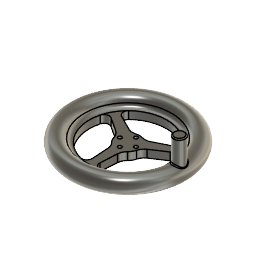
New+Assembly (Autodesk Fusion 360 archive; units mm, degrees)
design "handle"
Autodesk Fusion 360 part; units mm, degrees
note: some values were not read from the file. Set by a fixed rule: the direction of a hole.
sketch "Sketch1" plane through (0, 0, 0) normal (0, 1, 0) x (1, 0, 0)
  line L0 (0, 0) -> (50.8, 0)
  circle A0 centre (50.8, -8.255) radius 8.255
  line L1 (38.2276, -7.62) -> (0, -7.62)
  line L2 (0, -7.62) -> (0, 0)
  arc A1 (43.0171, -11.0067) -> (38.2276, -7.62) centre (38.2276, -12.7) ccw
  line L3 (45.085, -14.2118) -> (56.515, -14.2118)
  line L4 (56.515, -14.2118) -> (56.515, -39.6118)
  line L5 (56.515, -39.6118) -> (45.085, -39.6118)
  line L6 (45.085, -39.6118) -> (45.085, -14.2118)
  line L7 (50.8, -39.6118) -> (50.8, -14.2118)
  dimension "d1" = 16.51
  dimension "d2" = 7.62
  dimension "d3" = 5.08
  dimension "d4" = 50.8
  dimension "d6" = 25.4
  dimension "d20" = 11.43
  constraint coincident L0.start L2.end
  constraint horizontal L0
  constraint horizontal L1
  constraint vertical L2
  constraint tangent L0 A0
  constraint coincident L0.end A0
  constraint tangent A0 A1
  constraint coincident A0 A1.start
  constraint tangent L1 A1
  constraint horizontal L3
  constraint vertical L4
  constraint horizontal L5
  constraint vertical L6
  constraint coincident A0 L3.start
  constraint coincident A0 L3.end
  constraint midpoint L5 L7.start
  constraint midpoint L3 L7.end
  measures "d1" diameter of A0
  measures "d2" distance of L1.end L0.start
  measures "d3" radius of A1
  measures "d4" distance of A0.centre L2
  measures "d6" distance of L3.end L4.end
  measures "d20" distance of L3.start L3.end
revolve "Revolve1" add sketch "Sketch1" angle 360 about axis through (0, 0, 7.62) along (0, 0, -1) contours L0 A0 L1 L2 A1 | A0 L3 | A0 L3 L7 | A0 L3 L7
revolve "Revolve2" add sketch "Sketch1" angle 360 about axis through (50.8, 0, 39.6118) along (0, 0, -1) contours A0 L4 L5 L7 | A0 L3 L7 picked at (51.1497, -15.7216)
sketch "Sketch2" plane through (0, 0, 0) normal (0, 0, -1) x (1, 0, 0)
  circle A0 centre (0, 0) radius 50.8
  line L0 (0, 0) -> (50.8, 0)
  circle A1 centre (0, 0) radius 11.5
  circle A2 centre (0, 0) radius 38.2276
  line L1 (-5.08, 10.3172) -> (-3.429, 38.0735)
  line L2 (3.429, 38.0735) -> (5.08, 10.3172)
  line L3 (0, 0) -> (0, 8) construction
  line L4 (-6.3949, -9.558) -> (-31.2582, -22.0064)
  line L5 (-34.6872, -16.0672) -> (-11.4749, -0.7592)
  line L6 (11.4749, -0.7592) -> (34.6872, -16.0672)
  line L7 (31.2582, -22.0064) -> (6.3949, -9.558)
  point P0 (8, 0)
  point P1 (0, 8)
  point P2 (-8, 0)
  point P3 (0, -8)
  dimension "d9" = 8
  dimension "d11" = 360
  dimension "d12" = 23
  dimension "d13" = 6.858
  dimension "d14" = 10.16
  dimension "d16" = 360
  constraint coincident P0 L0
  constraint coincident A0.centre L0.start
  constraint coincident A1 L1.start
  constraint coincident A2 L1.end
  constraint coincident A2 L2.start
  constraint coincident P1 L3.end
  constraint symmetric L1 L2 L3
  constraint coincident A1 L2.end
  measures "d9" distance of P0 A0.centre
  measures "d12" diameter of A1
  measures "d13" distance of L1.end L2.start
  measures "d14" distance of L1.start L2.end
extrude "Extrude1" cut sketch "Sketch2" against normal through all contours L0 A1 A2 L2 | L0 A1 A2 L6 | A1 A2 L1 L5 | A1 A2 L4 L7
hole "Hole1" at (-8, 0, 0) at (0, -8, 0) at (8, 0, 0) at (0, 8, 0) direction (0, 0, 1) diameter 3.5992 end through all
fillet "Fillet1" radius 5.08 6 edges at (-34.6872, 16.0672, 3.81) (-31.2582, 22.0064, 3.81) (34.6872, 16.0672, 3.81) (31.2582, 22.0064, 3.81) (-3.429, -38.0735, 3.81) (3.429, -38.0735, 3.81)
fillet "Fillet1" radius 10.16 6 edges at (5.08, -10.3172, 3.81) (-5.08, -10.3172, 3.81) (-11.4749, 0.7592, 3.81) (-6.3949, 9.558, 3.81) (11.4749, 0.7592, 3.81) (6.3949, 9.558, 3.81)
fillet "Fillet1" radius 1.016 1 edges at (45.4717, -2.0666, 39.6118)
fillet "Fillet1" radius 1.016 2 edges at (50.6592, -5.7133, 16.508) (50.6414, 5.7128, 16.5084)

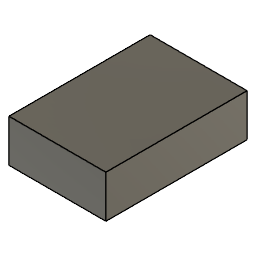
design "bread board w/ pico vol"
Autodesk Fusion 360 part; units mm, degrees
sketch "Sketch1" plane through (0, 0, 0) normal (0, 0, 1) x (1, 0, 0)
  line L0 (0, 0) -> (57, 0)
  line L1 (57, 0) -> (57, 83)
  line L2 (57, 83) -> (0, 83)
  line L3 (0, 83) -> (0, 0)
  dimension "d1" = 57
  dimension "d2" = 83
  constraint horizontal L0
  constraint vertical L1
  constraint horizontal L2
  constraint vertical L3
  constraint coincident L0.start L3.end
  measures "d1" distance of L0.start L0.end
  measures "d2" distance of L0.start L2.end
extrude "Extrude1" add sketch "Sketch1" along normal blind 25

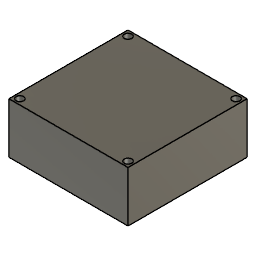
design "driver vol"
Autodesk Fusion 360 part; units mm, degrees
sketch "Sketch1" plane through (0, 0, 0) normal (0, 0, 1) x (1, 0, 0)
  line L0 (0, 0) -> (54, 0)
  line L1 (54, 0) -> (54, 54)
  line L2 (54, 54) -> (0, 54)
  line L3 (0, 54) -> (0, 0)
  line L4 (0, 54) -> (54, 0) construction
  point P0 (2.5, 51.5)
  point P1 (2.5, 2.5)
  point P2 (51.5, 51.5)
  point P3 (51.5, 2.5)
  dimension "d1" = 54
  dimension "d2" = 54
  dimension "d7" = 49
  dimension "d8" = 49
  dimension "d9" = 2.5
  constraint horizontal L0
  constraint vertical L1
  constraint horizontal L2
  constraint vertical L3
  constraint coincident L0.start L3.end
  constraint coincident P0 L4
  measures "d1" distance of L0.start L0.end
  measures "d2" distance of L0.start L2.end
  measures "d9" distance of L3 P0
extrude "Extrude1" add sketch "Sketch1" along normal blind 23
hole "Hole1" at (2.5, 2.5, 0) at (51.5, 2.5, 0) at (51.5, 51.5, 0) at (2.5, 51.5, 0) direction (0, 0, 1) diameter 3.4011 end through all
equation "d1 = d2"
equation "d2 = 49 mm + 5 mm"

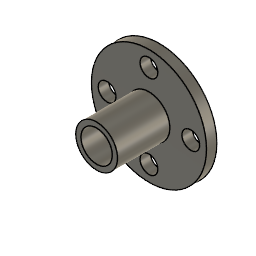
design "shaft flange"
Autodesk Fusion 360 part; units mm, degrees
sketch "Sketch1" plane through (0, 0, 0) normal (0, 1, 0) x (1, 0, 0)
  circle A0 centre (0, 0) radius 3
  circle A1 centre (0, 0) radius 4
  circle A2 centre (0, 0) radius 11
  point P0 (8, 0)
  point P1 (0, 8)
  point P2 (-8, 0)
  point P3 (0, -8)
  dimension "d1" = 6
  dimension "d2" = 8
  dimension "d3" = 22
  dimension "d4" = 8
  dimension "d6" = 360
  constraint coincident A0.centre A1.centre
  constraint concentric A0 A1
  constraint concentric A0 A2
  constraint horizontal A0.centre P0
  measures "d1" diameter of A0
  measures "d2" diameter of A1
  measures "d3" diameter of A2
  measures "d4" distance of A0.centre P0
extrude "Extrude1" add sketch "Sketch1" along normal blind 2 contours A1 | A2
extrude "Extrude2" add sketch "Sketch1" against normal blind 10 contours A1
hole "Hole1" at (8, 0, 0) at (0, 0, 8) at (-8, 0, 0) at (0, 0, -8) direction (0, 1, 0) diameter 3.4011 end through all
